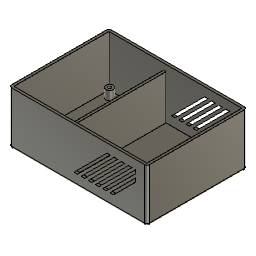
case (Autodesk Fusion 360 design; units mm, degrees)
Autodesk Fusion 360 part; units mm, degrees
sketch "Skizze1" plane through (0, 0, 0) normal (0, 0, 1) x (1, 0, 0)
  line L0 (0, 0) -> (105, 0)
  line L1 (105, 0) -> (105, 75)
  line L2 (105, 75) -> (0, 75)
  line L3 (0, 75) -> (0, 0)
  line L4 (0, 75.0065) -> (43, 75.0065) construction
  line L5 (43, 75) -> (45, 75)
  line L6 (45, 75) -> (45, 0)
  line L7 (45, 0) -> (43, 0)
  line L8 (43, 0) -> (43, 75)
  line L9 (45, 75.0065) -> (105, 75.0065) construction
  line L10 (0, 70) -> (43, 70) construction
  line L11 (0, 5) -> (43, 5) construction
  line L12 (2, 70) -> (2, 5) construction
  line L13 (2, 47.6883) -> (5.5, 47.6883) construction
  line L14 (5.5, 70) -> (5.5, 5) construction
  line L15 (35.5, 70) -> (35.5, 5) construction
  circle A0 centre (5.5, 70) radius 1.25
  circle A1 centre (5.5, 5) radius 1.25
  circle A2 centre (35.5, 70) radius 1.25
  circle A3 centre (35.5, 5) radius 1.25
  circle A4 centre (5.5, 70) radius 3
  circle A5 centre (35.5, 70) radius 3
  circle A6 centre (35.5, 5) radius 3
  circle A7 centre (5.5, 5) radius 3
  dimension "d1" = 105
  dimension "d2" = 75
  dimension "d7" = 43
  dimension "d8" = 2
  dimension "d9" = 75
  dimension "d31" = 60
  dimension "d33" = 5
  dimension "d45" = 3.5
  dimension "d47" = 2.5
  dimension "d48" = 2.5
  dimension "d49" = 2.5
  dimension "d50" = 2.5
  dimension "d51" = 6
  dimension "d52" = 6
  dimension "d53" = 6
  dimension "d54" = 6
  constraint horizontal L0
  constraint vertical L1
  constraint horizontal L2
  constraint vertical L3
  constraint coincident L0.start L3.end
  constraint coincident L3 L4.start
  constraint perpendicular L3 L4
  constraint horizontal L5
  constraint vertical L6
  constraint horizontal L7
  constraint vertical L8
  constraint coincident L2 L5.start
  constraint coincident L6 L9.start
  constraint coincident L1 L9.end
  constraint perpendicular L1 L9
  constraint coincident L8 L10.end
  constraint perpendicular L8 L10
  constraint coincident L3 L11.start
  constraint coincident L8 L11.end
  constraint perpendicular L8 L11
  constraint coincident L10 L12.start
  constraint coincident L11 L12.end
  constraint coincident L12 L13.start
  constraint perpendicular L12 L13
  constraint coincident L10 L14.start
  constraint coincident L11 L14.end
  constraint perpendicular L11 L14
  constraint coincident L10 L15.start
  constraint coincident L11 L15.end
  constraint perpendicular L11 L15
  constraint coincident L14.start A0.centre
  constraint coincident L14.end A1.centre
  constraint coincident L15.start A2.centre
  constraint coincident L15.end A3.centre
  constraint concentric A0 A4
  constraint concentric A1 A7
  measures "d1" distance of L0.start L0.end
  measures "d2" distance of L0.start L2.end
  measures "d7" distance of L4.start L4.end
  measures "d8" distance of L5.start L5.end
  measures "d9" distance of L5.start L7.end
  measures "d31" distance of L9.start L9.end
  measures "d33" distance of L2.end L10.start
  measures "d45" distance of L13.start L13.end
  measures "d47" diameter of A0
  measures "d48" diameter of A1
  measures "d49" diameter of A2
  measures "d50" diameter of A3
  measures "d51" diameter of A4
  measures "d52" diameter of A5
  measures "d53" diameter of A6
  measures "d54" diameter of A7
extrude "Extrusion1" add sketch "Skizze1" along normal blind 40 contours L0 L2 L3 L8 | L0 L2 L5 L6 L7 L8 | L0 L1 L2 L6 | A0 | A1 | A2 | A3 | A4 | A5 | A6 | A7
shell "Schale1" thickness 2 outward yes removed faces 1 at (85, 25, 40)
extrude "Extrusion2" add sketch "Skizze1" along normal blind 35 contours L0 L2 L5 L6 L7 L8
fillet "Abrundung1" radius 2 8 edges at (107, -2, 19) (107, 37.5, -2) (52.5, -2, -2) (-2, -2, 19) (107, 77, 19) (-2, 37.5, -2) (-2, 77, 19) (52.5, 77, -2)
sketch "Skizze2" plane through (0, -2, 0) normal (0, -1, 0) x (1, 0, 0)
  line L0 (105, 0) -> (105, 40)
  line L1 (105, 40) -> (0, 40)
  line L2 (0, 40) -> (0, 0)
  line L3 (0, 0) -> (105, 0)
  line L4 (105, 40) -> (45, 40) construction
  line L5 (105, 40) -> (65, 0)
  line L6 (105, 40) -> (161.5685, 40) construction
  line L7 (103.5858, 41.4142) -> (63.5858, 1.4142)
  line L8 (102.1716, 42.8284) -> (62.1716, 2.8284)
  line L9 (100.7574, 44.2426) -> (60.7574, 4.2426)
  line L10 (99.3431, 45.6569) -> (59.3431, 5.6569)
  line L11 (106.4142, 38.5858) -> (66.4142, -1.4142)
  line L12 (107.8284, 37.1716) -> (67.8284, -2.8284)
  line L13 (109.2426, 35.7574) -> (69.2426, -4.2426)
  line L14 (7, 7) -> (98, 7)
  line L15 (98, 7) -> (98, 33)
  line L16 (98, 33) -> (7, 33)
  line L17 (7, 33) -> (7, 7)
  line L18 (90.8579, 40) -> (50.8579, 0)
  line L19 (89.4437, 41.4142) -> (49.4437, 1.4142)
  line L20 (88.0294, 42.8284) -> (48.0294, 2.8284)
  line L21 (86.6152, 44.2426) -> (46.6152, 4.2426)
  dimension "d14" = 60
  dimension "d15" = 135
  dimension "d16" = 2
  dimension "d17" = 4
  dimension "d18" = 6
  dimension "d19" = 8
  dimension "d20" = -2
  dimension "d21" = -4
  dimension "d22" = -6
  dimension "d24" = -7
  dimension "d26" = 2
  dimension "d27" = 4
  dimension "d28" = 6
  constraint coincident L0.end L1.start
  constraint perpendicular L0 L4
  constraint horizontal L6
  constraint coincident L3 L5.end
  constraint coincident L1 L18.start
  constraint coincident L3 L18.end
  measures "d14" distance of L0.end L4.end
  measures "d15" angle of L5 L6
extrude "Extrusion3" cut sketch "Skizze2" against normal blind 110 contours L12 L13 L14 L15 | L5 L11 L14 L15 | L7 L8 L14 L16 | L14 L16 L18 L19 | L9 L10 L14 L16 | L14 L16 L20 L21
extrude "Extrusion4" add sketch "Skizze1" along normal blind 7 contours A7
extrude "Extrusion5" add sketch "Skizze1" along normal blind 7 contours A6
extrude "Extrusion6" add sketch "Skizze1" along normal blind 7 contours A4
extrude "Extrusion7" add sketch "Skizze1" along normal blind 7 contours A5
sketch "Skizze3" plane through (-2, 0, 0) normal (-1, 0, 0) x (0, -1, 0)
  line L0 (0, 0) -> (0, 40)
  line L1 (0, 40) -> (-75, 40)
  line L2 (-75, 40) -> (-75, 0)
  line L3 (-75, 0) -> (0, 0)
  line L4 (-75, 7) -> (0, 7) construction
  line L5 (-70, 0) -> (-70, 40) construction
  line L6 (-5, 0) -> (-5, 40) construction
  line L7 (-70, 7) -> (-16, 7) construction
  line L8 (-12.5, 8) -> (-19.5, 8) construction
  line L9 (-19.5, 8) -> (-19.5, 6) construction
  line L10 (-19.5, 6) -> (-12.5, 6) construction
  line L11 (-12.5, 6) -> (-12.5, 8) construction
  line L12 (-9.5, 11) -> (-22.5, 11)
  line L13 (-22.5, 11) -> (-22.5, 3)
  line L14 (-22.5, 3) -> (-9.5, 3)
  line L15 (-9.5, 3) -> (-9.5, 11)
  dimension "d66" = 54
  dimension "d72" = 7
  dimension "d73" = 2
  dimension "d74" = 3
  constraint coincident L2 L4.start
  constraint coincident L0 L4.end
  constraint perpendicular L0 L4
  constraint coincident L3 L5.start
  constraint coincident L1 L5.end
  constraint perpendicular L1 L5
  constraint coincident L3 L6.start
  constraint coincident L1 L6.end
  constraint perpendicular L1 L6
  constraint coincident L4 L7.start
  constraint coincident L5 L7.start
  constraint perpendicular L5 L7
  constraint horizontal L8
  constraint vertical L9
  constraint horizontal L10
  constraint vertical L11
  measures "d66" distance of L7.start L7.end
  measures "d72" distance of L8.start L8.end
  measures "d73" distance of L8.start L10.end
extrude "Extrusion8" cut sketch "Skizze3" against normal blind 8 contours L12 L13 L14 L15
